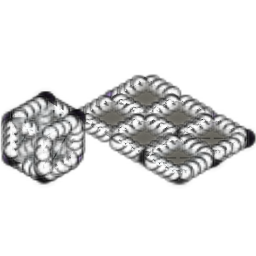
Kékesi Kristóf - Kocka v2 (Autodesk Fusion 360 design; units mm, degrees)
Autodesk Fusion 360 part; units mm, degrees
note: some values were not read from the file. Set by a fixed rule: which sketch regions a step uses.
sketch "Sketch1" plane through (0, 0, 0) normal (0, 0, 1) x (1, 0, 0) in component "Teli"
  line L0 (0, 0) -> (12.6, 0)
  line L1 (12.6, 0) -> (12.6, 4)
  line L2 (12.6, 4) -> (25.2, 4)
  line L3 (25.2, 4) -> (25.2, 0)
  line L4 (25.2, 0) -> (37.8, 0)
  line L5 (37.8, 0) -> (37.8, 4)
  line L6 (37.8, 4) -> (50.4, 4)
  line L7 (50.4, 4) -> (50.4, 0)
  line L8 (50.4, 0) -> (63, 0)
  line L9 (0, 63) -> (12.6, 63)
  line L10 (12.6, 63) -> (12.6, 59)
  line L11 (12.6, 59) -> (25.2, 59)
  line L12 (25.2, 59) -> (25.2, 63)
  line L13 (25.2, 63) -> (37.8, 63)
  line L14 (37.8, 63) -> (37.8, 59)
  line L15 (37.8, 59) -> (50.4, 59)
  line L16 (50.4, 59) -> (50.4, 63)
  line L17 (50.4, 63) -> (63, 63)
  line L18 (63, 63) -> (63, 50.4)
  line L19 (63, 50.4) -> (59, 50.4)
  line L20 (59, 50.4) -> (59, 37.8)
  line L21 (59, 37.8) -> (63, 37.8)
  line L22 (63, 37.8) -> (63, 25.2)
  line L23 (63, 25.2) -> (59, 25.2)
  line L24 (59, 25.2) -> (59, 12.6)
  line L25 (59, 12.6) -> (63, 12.6)
  line L26 (63, 12.6) -> (63, 0)
  line L27 (0, 63) -> (0, 50.4)
  line L28 (0, 50.4) -> (4, 50.4)
  line L29 (4, 50.4) -> (4, 37.8)
  line L30 (4, 37.8) -> (0, 37.8)
  line L31 (0, 37.8) -> (0, 25.2)
  line L32 (0, 25.2) -> (4, 25.2)
  line L33 (4, 25.2) -> (4, 12.6)
  line L34 (4, 12.6) -> (0, 12.6)
  line L35 (0, 12.6) -> (0, 0)
  line L36 (12.7, 65) -> (12.7, 61)
  line L37 (25.1, 61) -> (25.1, 65)
  line L38 (37.9, 65) -> (37.9, 61)
  line L39 (50.3, 61) -> (50.3, 65)
  line L40 (65, 50.3) -> (61, 50.3)
  line L41 (61, 37.9) -> (65, 37.9)
  line L42 (65, 25.1) -> (61, 25.1)
  line L43 (61, 12.7) -> (65, 12.7)
  line L44 (50.3, 4) -> (50.3, 0)
  line L45 (37.9, 0) -> (37.9, 4)
  line L46 (25.1, 4) -> (25.1, 0)
  line L47 (12.7, 0) -> (12.7, 4)
  line L48 (4, 12.7) -> (0, 12.7)
  line L49 (0, 25.1) -> (4, 25.1)
  line L50 (4, 37.9) -> (0, 37.9)
  line L51 (0, 50.3) -> (4, 50.3)
  dimension "d1" = 63
  dimension "d2" = 63
  dimension "d3" = 4
  dimension "d8" = 4
  dimension "d9" = 4
  dimension "d10" = 4
  dimension "d88" = -0.1
  dimension "d89" = -0.1
  dimension "d90" = -0.1
  dimension "d91" = -0.1
  dimension "d92" = -0.1
  dimension "d93" = -0.1
  dimension "d94" = -0.1
  dimension "d95" = -0.1
  dimension "d96" = 0.1
  dimension "d97" = 0.1
  dimension "d98" = 0.1
  dimension "d99" = 0.1
  dimension "d100" = 0.1
  dimension "d101" = 0.1
  dimension "d102" = 0.1
  dimension "d103" = 0.1
  constraint coincident L0.start L35.end
  constraint perpendicular L0 L1
  constraint perpendicular L1 L2
  constraint perpendicular L2 L3
  constraint perpendicular L3 L4
  constraint perpendicular L4 L5
  constraint perpendicular L3 L6
  constraint perpendicular L4 L7
  constraint equal L0 L2
  constraint equal L2 L4
  constraint equal L4 L6
  constraint equal L6 L8
  constraint collinear L2 L6
  constraint collinear L4 L8
  constraint collinear L0 L8
  constraint perpendicular L9 L10
  constraint perpendicular L10 L11
  constraint perpendicular L11 L12
  constraint perpendicular L12 L13
  constraint perpendicular L13 L14
  constraint perpendicular L14 L15
  constraint perpendicular L15 L16
  constraint horizontal L2
  constraint equal L9 L11
  constraint equal L11 L13
  constraint equal L13 L15
  constraint equal L15 L17
  constraint collinear L13 L17
  constraint collinear L9 L13
  constraint collinear L11 L15
  constraint perpendicular L17 L18
  constraint perpendicular L18 L19
  constraint perpendicular L19 L20
  constraint perpendicular L20 L21
  constraint perpendicular L21 L22
  constraint perpendicular L22 L23
  constraint perpendicular L23 L24
  constraint perpendicular L24 L25
  constraint perpendicular L8 L26
  constraint equal L18 L20
  constraint equal L20 L22
  constraint equal L22 L24
  constraint equal L24 L26
  constraint collinear L18 L22
  constraint collinear L22 L26
  constraint collinear L20 L24
  constraint perpendicular L9 L27
  constraint perpendicular L27 L28
  constraint perpendicular L9 L29
  constraint perpendicular L29 L30
  constraint perpendicular L30 L31
  constraint perpendicular L31 L32
  constraint perpendicular L32 L33
  constraint perpendicular L33 L34
  constraint vertical L35
  constraint equal L27 L29
  constraint equal L29 L31
  constraint equal L31 L33
  constraint equal L33 L35
  constraint collinear L27 L31
  constraint collinear L31 L35
  constraint collinear L29 L33
  measures "d1" distance of L9.start L17.end
  measures "d2" distance of L0.start L9.start
  measures "d3" distance of L0.end L1.end
  measures "d8" distance of L13.end L14.end
  measures "d9" distance of L18.end L19.end
  measures "d10" distance of L27.end L28.end
extrude "Extrude1" add sketch "Sketch1" along normal blind 4 makes body 1 in component "Teli"
sketch "Sketch2" plane through (0, 0, 0) normal (0, 0, 1) x (1, 0, 0) in component "Feles"
  line L0 (-63, -55) -> (-50.4, -55)
  line L1 (-50.4, -55) -> (-50.4, -59)
  line L2 (-50.4, -59) -> (-37.8, -59)
  line L3 (-37.8, -59) -> (-37.8, -55)
  line L4 (-37.8, -55) -> (-25.2, -55)
  line L5 (-25.2, -55) -> (-25.2, -59)
  line L6 (-25.2, -59) -> (-12.6, -59)
  line L7 (-12.6, -59) -> (-12.6, -55)
  line L8 (-12.6, -55) -> (0, -55)
  line L9 (-63, 0) -> (-50.4, 0)
  line L10 (-50.4, 0) -> (-50.4, 4)
  line L11 (-50.4, 4) -> (-37.8, 4)
  line L12 (-37.8, 4) -> (-37.8, 0)
  line L13 (-37.8, 0) -> (-25.2, 0)
  line L14 (-25.2, 0) -> (-25.2, 4)
  line L15 (-25.2, 4) -> (-12.6, 4)
  line L16 (-12.6, 4) -> (-12.6, 0)
  line L17 (-12.6, 0) -> (0, 0)
  line L18 (-12.6, -59) -> (0, -59) construction
  line L19 (0, 4) -> (-12.6, 4) construction
  line L20 (0, -55) -> (0, -46.4)
  line L21 (0, -46.4) -> (-4, -46.4)
  line L22 (-4, -46.4) -> (-4, -33.8)
  line L23 (-4, -33.8) -> (0, -33.8)
  line L24 (0, -21.2) -> (-4, -21.2)
  line L25 (-4, -21.2) -> (-4, -8.6)
  line L26 (-4, -8.6) -> (0, -8.6)
  line L27 (0, -8.6) -> (0, 0)
  line L28 (0, -33.8) -> (0, -21.2)
  line L29 (0, -59) -> (0, -46.4) construction
  line L30 (0, 4) -> (0, -8.6) construction
  line L31 (-63, -55) -> (-63, -46.4)
  line L32 (-63, -46.4) -> (-59, -46.4)
  line L33 (-59, -46.4) -> (-59, -33.8)
  line L34 (-59, -33.8) -> (-63, -33.8)
  line L35 (-63, -33.8) -> (-63, -21.2)
  line L36 (-63, -21.2) -> (-59, -21.2)
  line L37 (-59, -21.2) -> (-59, -8.6)
  line L38 (-59, -8.6) -> (-63, -8.6)
  line L39 (-63, -8.6) -> (-63, 0)
  line L40 (-50.5, 0) -> (-50.5, 4)
  line L41 (-37.7, 4) -> (-37.7, 0)
  line L42 (-25.3, 0) -> (-25.3, 4)
  line L43 (-12.5, 4) -> (-12.5, 0)
  line L44 (-4, -8.7) -> (0, -8.7)
  line L45 (0, -21.1) -> (-4, -21.1)
  line L46 (-4, -33.9) -> (0, -33.9)
  line L47 (0, -46.3) -> (-4, -46.3)
  line L48 (-12.5, -61) -> (-12.5, -57)
  line L49 (-25.3, -57) -> (-25.3, -61)
  line L50 (-37.7, -61) -> (-37.7, -57)
  line L51 (-50.5, -57) -> (-50.5, -61)
  line L52 (-65, -46.3) -> (-61, -46.3)
  line L53 (-61, -33.9) -> (-65, -33.9)
  line L54 (-65, -21.1) -> (-61, -21.1)
  line L55 (-61, -8.7) -> (-65, -8.7)
  dimension "d15" = 63
  dimension "d17" = 4
  dimension "d18" = 4
  dimension "d61" = 63
  dimension "d62" = 4
  dimension "d87" = 4
  dimension "d104" = -0.1
  dimension "d105" = -0.1
  dimension "d106" = -0.1
  dimension "d107" = -0.1
  dimension "d108" = 0.1
  dimension "d109" = 0.1
  dimension "d110" = 0.1
  dimension "d111" = 0.1
  dimension "d112" = 0.1
  dimension "d113" = 0.1
  dimension "d114" = 0.1
  dimension "d115" = 0.1
  dimension "d116" = -0.1
  dimension "d117" = -0.1
  dimension "d118" = -0.1
  dimension "d119" = -0.1
  constraint coincident L17.end L27.end
  constraint perpendicular L0 L1
  constraint perpendicular L1 L2
  constraint perpendicular L2 L3
  constraint perpendicular L3 L4
  constraint perpendicular L4 L5
  constraint perpendicular L5 L6
  constraint perpendicular L6 L7
  constraint horizontal L8
  constraint equal L6 L8
  constraint equal L4 L6
  constraint equal L2 L4
  constraint equal L0 L2
  constraint collinear L0 L4
  constraint collinear L4 L8
  constraint collinear L2 L6
  constraint perpendicular L9 L10
  constraint perpendicular L10 L11
  constraint perpendicular L11 L12
  constraint perpendicular L12 L13
  constraint perpendicular L13 L14
  constraint perpendicular L14 L15
  constraint perpendicular L15 L16
  constraint horizontal L17
  constraint collinear L9 L13
  constraint collinear L13 L17
  constraint collinear L11 L15
  constraint equal L13 L15
  constraint equal L15 L17
  constraint perpendicular L7 L18
  constraint horizontal L19
  constraint perpendicular L8 L20
  constraint perpendicular L20 L21
  constraint perpendicular L21 L22
  constraint perpendicular L17 L27
  constraint horizontal L24
  constraint horizontal L23
  constraint horizontal L26
  constraint perpendicular L24 L28
  constraint perpendicular L21 L29
  constraint perpendicular L26 L30
  constraint equal L25 L30
  constraint equal L25 L28
  constraint equal L22 L28
  constraint equal L22 L29
  constraint collinear L22 L25
  constraint collinear L20 L28
  constraint collinear L28 L30
  constraint collinear L5 L14
  constraint collinear L1 L10
  constraint perpendicular L0 L31
  constraint perpendicular L31 L32
  constraint perpendicular L0 L33
  constraint perpendicular L33 L34
  constraint perpendicular L0 L35
  constraint perpendicular L35 L36
  constraint perpendicular L0 L37
  constraint perpendicular L37 L38
  constraint vertical L39
  constraint collinear L33 L37
  constraint collinear L35 L39
  constraint collinear L31 L35
  constraint collinear L26 L38
  constraint collinear L24 L36
  constraint collinear L23 L34
  constraint collinear L21 L32
  measures "d15" distance of L17.end L9.start
  measures "d17" distance of L2.end L3.end
  measures "d18" distance of L11.end L12.end
  measures "d61" distance of L18.end L19.start
  measures "d62" distance of L20.end L21.end
  measures "d87" distance of L33.end L34.end
extrude "Extrude2" add sketch "Sketch2" along normal blind 4 separate body makes body 2 in component "Feles"
sketch "Sketch2 (2)" plane through (0, 0, 0) normal (0, 0, 1) x (1, 0, 0) in component "Üres"
  line L0 (0, 0) -> (-63, 0) construction
  line L1 (-63, 0) -> (-63, -63) construction
  line L2 (-63, -63) -> (0, -63) construction
  line L3 (0, -63) -> (0, 0) construction
  line L4 (-59, -59) -> (-63, -59) construction
  line L5 (-59, -59) -> (-59, -63) construction
  line L6 (-4, -4) -> (-4, 0) construction
  line L7 (-59, -63) -> (-59, -50.4) construction
  line L8 (-59, -50.4) -> (-63, -50.4)
  line L9 (-63, -37.8) -> (-59, -37.8)
  line L10 (-59, -37.8) -> (-59, -25.2)
  line L11 (-63, -25.2) -> (-63, -12.6)
  line L12 (-59, -12.6) -> (-59, 0) construction
  line L13 (-63, -25.2) -> (-59, -25.2)
  line L14 (-63, -12.6) -> (-59, -12.6)
  line L15 (-63, -50.4) -> (-63, -37.8)
  line L16 (-59, -59) -> (-59, -50.4)
  line L17 (-59, -37.8) -> (-59, -25.2)
  line L18 (-59, -12.6) -> (-59, -4)
  line L19 (-4, -4) -> (-12.6, -4)
  line L20 (-12.6, -4) -> (-12.6, 0)
  line L21 (-12.6, 0) -> (-25.2, 0)
  line L22 (-25.2, -4) -> (-37.8, -4)
  line L23 (-37.8, -4) -> (-37.8, 0)
  line L24 (-50.4, 0) -> (-50.4, -4)
  line L25 (-50.4, -4) -> (-59, -4)
  line L26 (-50.4, 0) -> (-37.8, 0)
  line L27 (-25.2, -4) -> (-25.2, 0)
  line L28 (0, -4) -> (-12.6, -4) construction
  line L29 (-63, -4) -> (-50.4, -4) construction
  line L30 (-4, -4) -> (0, -4) construction
  line L31 (-59, -59) -> (-4, -4) construction
  line L32 (-59, -59) -> (-4, -4) construction
  line L33 (-4, -4) -> (-4, 0) construction
  line L34 (0, -12.6) -> (0, -25.2)
  line L35 (-4, 0) -> (-4, -12.6) construction
  line L36 (-4, -25.2) -> (0, -25.2)
  line L37 (-37.8, -63) -> (-37.8, -59)
  line L38 (-63, -59) -> (-50.4, -59) construction
  line L39 (-4, -12.6) -> (0, -12.6)
  line L40 (-4, -37.8) -> (0, -37.8)
  line L41 (-50.4, -59) -> (-50.4, -63)
  line L42 (0, -50.4) -> (0, -37.8)
  line L43 (-59, -59) -> (-50.4, -59)
  line L44 (0, -50.4) -> (-4, -50.4)
  line L45 (-4, -4) -> (-4, -12.6)
  line L46 (-12.6, -59) -> (-4, -59)
  line L47 (0, 0) -> (0, -63) construction
  line L48 (-4, -50.4) -> (-4, -59)
  line L49 (-12.6, -63) -> (-12.6, -59)
  line L50 (-4, -25.2) -> (-4, -37.8)
  line L51 (-37.8, -59) -> (-25.2, -59)
  line L52 (-4, -4) -> (0, -4) construction
  line L53 (0, -63) -> (-63, -63) construction
  line L54 (-12.6, -59) -> (0, -59) construction
  line L55 (-25.2, -63) -> (-12.6, -63)
  line L56 (-4, -63) -> (-4, -50.4) construction
  line L57 (-50.4, -63) -> (-37.8, -63)
  line L58 (-37.8, -59) -> (-25.2, -59)
  line L59 (-25.2, -63) -> (-25.2, -59)
  line L60 (-50.5, 0) -> (-50.5, -4)
  line L61 (-37.7, -4) -> (-37.7, 0)
  line L62 (-25.3, -4) -> (-25.3, 0)
  line L63 (-12.5, -4) -> (-12.5, 0)
  line L64 (-4, -12.5) -> (0, -12.5)
  line L65 (-4, -25.3) -> (0, -25.3)
  line L66 (-4, -37.7) -> (0, -37.7)
  line L67 (0, -50.5) -> (-4, -50.5)
  line L68 (-12.5, -65) -> (-12.5, -61)
  line L69 (-25.3, -65) -> (-25.3, -61)
  line L70 (-37.7, -65) -> (-37.7, -61)
  line L71 (-50.5, -61) -> (-50.5, -65)
  line L72 (-61, -50.5) -> (-65, -50.5)
  line L73 (-65, -37.7) -> (-61, -37.7)
  line L74 (-65, -25.3) -> (-61, -25.3)
  line L75 (-65, -12.5) -> (-61, -12.5)
  dimension "d48" = 63
  dimension "d49" = 63
  dimension "d50" = 4
  dimension "d51" = 4
  dimension "d53" = 4
  dimension "d54" = 4
  dimension "d120" = 0.1
  dimension "d121" = 0.1
  dimension "d122" = -0.1
  dimension "d123" = 0.1
  dimension "d124" = -0.1
  dimension "d125" = 0.1
  dimension "d126" = -0.1
  dimension "d127" = -0.1
  dimension "d128" = 0.1
  dimension "d129" = -0.1
  dimension "d130" = 0.1
  dimension "d131" = 0.1
  dimension "d132" = -0.1
  dimension "d133" = -0.1
  dimension "d134" = 0.1
  dimension "d135" = -0.1
  constraint horizontal L0
  constraint vertical L1
  constraint horizontal L2
  constraint vertical L3
  constraint coincident L0.start L3.end
  constraint vertical L16
  constraint coincident L1 L4.end
  constraint perpendicular L1 L4
  constraint coincident L2 L5.end
  constraint perpendicular L2 L5
  constraint coincident L0 L6.end
  constraint perpendicular L0 L6
  constraint coincident L1 L8.end
  constraint perpendicular L1 L8
  constraint coincident L1 L9.start
  constraint coincident L9.end L16
  constraint perpendicular L9 L16
  constraint coincident L10.end L16
  constraint coincident L1 L11.start
  constraint coincident L1 L11.end
  constraint coincident L12.start L16
  constraint coincident L0 L12.end
  constraint perpendicular L0 L12
  constraint perpendicular L13 L16
  constraint perpendicular L14 L16
  constraint equal L7 L15
  constraint equal L10 L15
  constraint equal L10 L11
  constraint equal L11 L12
  constraint collinear L16 L17
  constraint collinear L17 L18
  constraint coincident L0 L20.end
  constraint perpendicular L0 L20
  constraint coincident L0 L21.end
  constraint perpendicular L20 L22
  constraint coincident L0 L23.end
  constraint perpendicular L0 L23
  constraint coincident L0 L24.start
  constraint perpendicular L0 L24
  constraint perpendicular L21 L27
  constraint collinear L19 L22
  constraint collinear L22 L25
  constraint coincident L3 L28.start
  constraint coincident L1 L29.start
  constraint equal L26 L29
  constraint equal L22 L26
  constraint equal L21 L22
  constraint equal L21 L28
  constraint horizontal L29
  constraint horizontal L28
  constraint symmetric L0.start L31 L3.end
  constraint symmetric L0.end L31 L2.end
  constraint symmetric L1.end L31 L2.start
  constraint symmetric L4.start L31 L5.start
  constraint symmetric L18.end L31 L46.end
  constraint symmetric L6.start L31 L19.start
  constraint symmetric L5.end L31 L4.end
  constraint symmetric L6.end L31 L28.start
  constraint symmetric L7.end L31 L38.end
  constraint symmetric L8.end L31 L41.end
  constraint symmetric L9.start L31 L37.start
  constraint symmetric L9.end L31 L37.end
  constraint symmetric L10.end L31 L51.end
  constraint symmetric L11.start L31 L55.start
  constraint symmetric L11.end L31 L49.start
  constraint symmetric L12.start L31 L46.start
  constraint symmetric L12.end L31 L54.end
  constraint symmetric L19.end L31 L35.end
  constraint symmetric L20.end L31 L34.start
  constraint symmetric L21.end L31 L34.end
  constraint symmetric L22.start L31 L36.start
  constraint symmetric L22.end L31 L40.start
  constraint symmetric L23.end L31 L40.end
  constraint symmetric L24.start L31 L42.start
  constraint symmetric L24.end L31 L44.end
  constraint symmetric L28.start L31 L6.end
  constraint symmetric L29.start L31 L56.start
  measures "d48" distance of L0.start L0.end
  measures "d49" distance of L0.start L2.end
  measures "d50" distance of L4.start L4.end
  measures "d51" distance of L4.start L5.end
  measures "d53" distance of L6.start L6.end
  measures "d54" distance of L6.start L28.start
extrude "Extrude2'" add sketch "Sketch2 (2)" along normal blind 4 separate body makes body 3 in component "Üres"
other "Arrange1"
component "Feles" placed x (1, 0, 0) y (0, 0, -1) z (0, 1, 0) at (63, 0, 4)
component "Üres" placed x (0, 0, 1) y (0, 1, 0) z (-1, 0, 0) at (63, 63, 63)
component "Feles" placed x (1, 0, 0) y (0, 0, -1) z (0, 1, 0) at (63, 59, 4)
component "Üres" placed x (0, 0, 1) y (0, 1, 0) z (-1, 0, 0) at (4, 63, 63)
component "Teli" placed x (1, 0, 0) y (0, 1, 0) z (0, 0, 1) at (0, 0, 0)
component "Teli" placed x (1, 0, 0) y (0, 1, 0) z (0, 0, 1) at (0, 0, 59)
component "Arrange1" placed x (1, 0, 0) y (0, 1, 0) z (0, 0, 1) at (0, 0, 0)
component "Envelope1(Qty: 1)" placed x (1, 0, 0) y (0, 1, 0) z (0, 0, 1) at (0, 125, 0) in component "Arrange1"
component "Teli" placed x (1, 0, 0) y (0, 1, 0) z (0, 0, 1) at (2, 2, 0) in component "Envelope1(Qty: 1)"
component "Feles" placed x (1, 0, 0) y (0, 1, 0) z (0, 0, 1) at (130, 61, 0) in component "Envelope1(Qty: 1)"
component "Üres" placed x (1, 0, 0) y (0, 1, 0) z (0, 0, 1) at (195, 65, 0) in component "Envelope1(Qty: 1)"
component "Teli" placed x (1, 0, 0) y (0, 1, 0) z (0, 0, 1) at (2, 67, 0) in component "Envelope1(Qty: 1)"
component "Feles" placed x (1, 0, 0) y (0, 1, 0) z (0, 0, 1) at (130, 126, 0) in component "Envelope1(Qty: 1)"
component "Üres" placed x (1, 0, 0) y (0, 1, 0) z (0, 0, 1) at (195, 130, 0) in component "Envelope1(Qty: 1)"
equation "d2 = d1"
equation "d6 = d3"
equation "d8 = d3"
equation "d9 = d3"
equation "d10 = d3"
equation "d15 = d1"
equation "d17 = d3"
equation "d18 = d3"
equation "d19 = d3"
equation "d48 = d1"
equation "d49 = d1"
equation "d50 = d3"
equation "d51 = d3"
equation "d53 = d3"
equation "d54 = d3"
equation "d55 = d3"
equation "d61 = d1"
equation "d62 = d3"
equation "d87 = d3"
